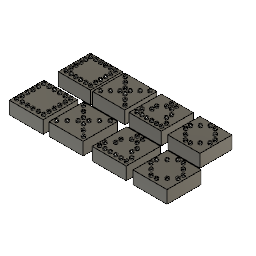
BrailleResearchShapes (Autodesk Fusion 360 design; units mm, degrees)
Autodesk Fusion 360 part; units mm, degrees
(part 1 of 2)
sketch "Sketch1" plane through (0, 0, 0) normal (0, 0, 1) x (1, 0, 0)
  circle A0 centre (3.4, 9.3) radius 0.75
  circle A1 centre (5.7, 9.2955) radius 0.75
  circle A2 centre (3.4, 7) radius 0.75
  circle A3 centre (5.7, 7) radius 0.75
  circle A4 centre (3.4, 4.7) radius 0.75
  circle A5 centre (5.7, 4.7) radius 0.75
  circle A6 centre (8, 9.3) radius 0.75
  circle A7 centre (10.3, 9.2955) radius 0.75
  circle A8 centre (10.3, 7) radius 0.75
  circle A9 centre (8, 7) radius 0.75
  circle A10 centre (10.3, 4.7) radius 0.75
  circle A11 centre (8, 4.7) radius 0.75
  circle A12 centre (12.6, 9.3) radius 0.75
  circle A13 centre (14.9, 7) radius 0.75
  circle A14 centre (14.9, 9.2955) radius 0.75
  circle A15 centre (12.6, 7) radius 0.75
  circle A16 centre (12.6, 4.7) radius 0.75
  circle A17 centre (14.9, 4.7) radius 0.75
  circle A18 centre (3.4, 2.4) radius 0.75
  circle A19 centre (5.7, 2.3955) radius 0.75
  circle A20 centre (5.7, 0.1) radius 0.75
  circle A21 centre (8, 0) radius 0.75
  circle A22 centre (8, 2.3) radius 0.75
  circle A23 centre (3.4, 0.1) radius 0.75
  circle A24 centre (10.3, 2.2955) radius 0.75
  circle A25 centre (5.7, -2.2) radius 0.75
  circle A26 centre (12.6, 2.3) radius 0.75
  circle A27 centre (12.6, 0) radius 0.75
  circle A28 centre (10.3, -2.3) radius 0.75
  circle A29 centre (10.3, 0) radius 0.75
  circle A30 centre (3.4, -2.2) radius 0.75
  circle A31 centre (8, -2.3) radius 0.75
  circle A32 centre (14.9, 0) radius 0.75
  circle A33 centre (12.6, -2.3) radius 0.75
  circle A34 centre (14.9, -2.3) radius 0.75
  circle A35 centre (14.9, 2.2955) radius 0.75
  line L0 (1.5, 11) -> (16.5, 11)
  line L1 (16.5, 11) -> (16.5, -4)
  line L2 (16.5, -4) -> (1.5, -4)
  line L3 (1.5, -4) -> (1.5, 11)
  line L4 (17.5, 11) -> (32.5, 11)
  circle A36 centre (28.6, 9.3) radius 0.75
  circle A37 centre (26.3, 9.2955) radius 0.75
  circle A38 centre (24, 7) radius 0.75
  circle A39 centre (21.7, 9.2955) radius 0.75
  circle A40 centre (19.4, 9.3) radius 0.75
  circle A41 centre (19.4, 7) radius 0.75
  circle A42 centre (21.7, 7) radius 0.75
  circle A43 centre (28.6, 7) radius 0.75
  circle A44 centre (30.9, 7) radius 0.75
  line L5 (32.5, 11) -> (32.5, -4)
  circle A45 centre (30.9, 2.2955) radius 0.75
  circle A46 centre (30.9, 0) radius 0.75
  circle A47 centre (30.9, -2.3) radius 0.75
  line L6 (32.5, -4) -> (17.5, -4)
  line L7 (17.5, -4) -> (17.5, 11)
  circle A48 centre (19.4, 2.4) radius 0.75
  circle A49 centre (21.7, 2.3955) radius 0.75
  circle A50 centre (19.4, 4.7) radius 0.75
  circle A51 centre (24, 9.3) radius 0.75
  circle A52 centre (21.7, 4.7) radius 0.75
  circle A53 centre (24, 4.7) radius 0.75
  circle A54 centre (24, 2.3) radius 0.75
  circle A55 centre (26.3, 7) radius 0.75
  circle A56 centre (30.9, 9.2955) radius 0.75
  circle A57 centre (28.6, 4.7) radius 0.75
  circle A58 centre (26.3, 4.7) radius 0.75
  circle A59 centre (26.3, 2.2955) radius 0.75
  circle A60 centre (30.9, 4.7) radius 0.75
  circle A61 centre (28.6, 2.3) radius 0.75
  circle A62 centre (28.6, 0) radius 0.75
  circle A63 centre (26.3, 0) radius 0.75
  circle A64 centre (26.3, -2.3) radius 0.75
  circle A65 centre (28.6, -2.3) radius 0.75
  circle A66 centre (21.7, 0.1) radius 0.75
  circle A67 centre (24, 0) radius 0.75
  circle A68 centre (24, -2.3) radius 0.75
  circle A69 centre (21.7, -2.2) radius 0.75
  circle A70 centre (19.4, 0.1) radius 0.75
  circle A71 centre (19.4, -2.2) radius 0.75
  line L8 (34.5, 11) -> (49.5, 11)
  line L9 (49.5, 11) -> (49.5, -4)
  circle A72 centre (47.9, 9.2955) radius 0.75
  circle A73 centre (45.6, 9.3) radius 0.75
  circle A74 centre (45.6, 7) radius 0.75
  circle A75 centre (45.6, 4.7) radius 0.75
  circle A76 centre (45.6, 2.3) radius 0.75
  circle A77 centre (45.6, 0) radius 0.75
  circle A78 centre (45.6, -2.3) radius 0.75
  line L10 (49.5, -4) -> (34.5, -4)
  circle A79 centre (41, -2.3) radius 0.75
  circle A80 centre (38.7, -2.2) radius 0.75
  circle A81 centre (36.4, -2.2) radius 0.75
  line L11 (34.5, -4) -> (34.5, 11)
  circle A82 centre (36.4, 0.1) radius 0.75
  circle A83 centre (38.7, 2.3955) radius 0.75
  circle A84 centre (36.4, 2.4) radius 0.75
  circle A85 centre (36.4, 4.7) radius 0.75
  circle A86 centre (36.4, 7) radius 0.75
  circle A87 centre (36.4, 9.3) radius 0.75
  circle A88 centre (38.7, 9.2955) radius 0.75
  circle A89 centre (41, 9.3) radius 0.75
  circle A90 centre (43.3, 9.2955) radius 0.75
  circle A91 centre (43.3, 7) radius 0.75
  circle A92 centre (41, 7) radius 0.75
  circle A93 centre (41, 4.7) radius 0.75
  circle A94 centre (38.7, 7) radius 0.75
  circle A95 centre (38.7, 4.7) radius 0.75
  circle A96 centre (43.3, 4.7) radius 0.75
  circle A97 centre (47.9, 7) radius 0.75
  circle A98 centre (47.9, 4.7) radius 0.75
  circle A99 centre (47.9, 2.2955) radius 0.75
  circle A100 centre (47.9, 0) radius 0.75
  circle A101 centre (47.9, -2.3) radius 0.75
  circle A102 centre (43.3, -2.3) radius 0.75
  circle A103 centre (43.3, 0) radius 0.75
  circle A104 centre (43.3, 2.2955) radius 0.75
  circle A105 centre (41, 0) radius 0.75
  circle A106 centre (41, 2.3) radius 0.75
  circle A107 centre (38.7, 0.1) radius 0.75
  circle A108 centre (3.2346, -12.4941) radius 0.75
  circle A109 centre (5.7346, -12.4941) radius 0.75
  circle A110 centre (5.7346, -14.9941) radius 0.75
  circle A111 centre (3.2346, -14.9941) radius 0.75
  circle A112 centre (3.2346, -17.4941) radius 0.75
  circle A113 centre (5.7346, -17.4941) radius 0.75
  circle A114 centre (8.2346, -12.4941) radius 0.75
  circle A115 centre (10.7346, -14.9941) radius 0.75
  circle A116 centre (10.7346, -17.4941) radius 0.75
  circle A117 centre (8.2346, -17.4941) radius 0.75
  circle A118 centre (8.2346, -14.9941) radius 0.75
  circle A119 centre (10.7346, -12.4941) radius 0.75
  circle A120 centre (13.2346, -12.4941) radius 0.75
  circle A121 centre (13.2346, -14.9941) radius 0.75
  circle A122 centre (13.2346, -17.4941) radius 0.75
  circle A123 centre (15.7346, -17.4941) radius 0.75
  circle A124 centre (15.7346, -14.9941) radius 0.75
  circle A125 centre (15.7346, -12.4941) radius 0.75
  circle A126 centre (3.2346, -19.9941) radius 0.75
  circle A127 centre (5.7346, -19.9941) radius 0.75
  circle A128 centre (8.2346, -22.4941) radius 0.75
  circle A129 centre (5.7346, -24.9941) radius 0.75
  circle A130 centre (5.7346, -22.4941) radius 0.75
  circle A131 centre (8.2346, -19.9941) radius 0.75
  circle A132 centre (3.2346, -22.4941) radius 0.75
  circle A133 centre (3.2346, -24.9941) radius 0.75
  circle A134 centre (10.7346, -19.9941) radius 0.75
  circle A135 centre (10.7346, -22.4941) radius 0.75
  circle A136 centre (8.2346, -24.9941) radius 0.75
  circle A137 centre (10.7346, -24.9941) radius 0.75
  circle A138 centre (13.2346, -19.9941) radius 0.75
  circle A139 centre (15.7346, -19.9941) radius 0.75
  circle A140 centre (13.2346, -22.4941) radius 0.75
  circle A141 centre (13.2346, -24.9941) radius 0.75
  circle A142 centre (15.7346, -22.4941) radius 0.75
  circle A143 centre (15.7346, -24.9941) radius 0.75
  line L12 (17.4146, -10.7288) -> (17.4146, -26.9182)
  line L13 (1.5963, -10.7288) -> (17.4146, -10.7288)
  line L14 (17.4146, -26.9182) -> (1.5963, -26.9182)
  line L15 (1.5963, -26.9182) -> (1.5963, -10.7288)
  line L16 (19.5963, -10.2888) -> (35.4146, -10.2888)
  line L17 (19.5963, -26.3316) -> (19.5963, -10.2888)
  circle A144 centre (21.2346, -11.9941) radius 0.75
  circle A145 centre (23.7346, -11.9941) radius 0.75
  circle A146 centre (21.2346, -16.9941) radius 0.75
  circle A147 centre (23.7346, -14.4941) radius 0.75
  circle A148 centre (26.2346, -11.9941) radius 0.75
  circle A149 centre (26.2346, -14.4941) radius 0.75
  circle A150 centre (23.7346, -16.9941) radius 0.75
  circle A151 centre (21.2346, -21.9941) radius 0.75
  circle A152 centre (23.7346, -19.4941) radius 0.75
  circle A153 centre (28.7346, -14.4941) radius 0.75
  circle A154 centre (26.2346, -16.9941) radius 0.75
  circle A155 centre (23.7346, -21.9941) radius 0.75
  circle A156 centre (28.7346, -16.9941) radius 0.75
  circle A157 centre (33.7346, -11.9941) radius 0.75
  circle A158 centre (31.2346, -14.4941) radius 0.75
  circle A159 centre (26.2346, -19.4941) radius 0.75
  line L18 (35.4146, -26.3316) -> (19.5963, -26.3316)
  circle A160 centre (23.7346, -24.4941) radius 0.75
  line L19 (35.4146, -10.2888) -> (35.4146, -26.3316)
  circle A161 centre (33.7346, -19.4941) radius 0.75
  circle A162 centre (31.2346, -24.4941) radius 0.75
  circle A163 centre (28.7346, -19.4941) radius 0.75
  circle A164 centre (33.7346, -14.4941) radius 0.75
  circle A165 centre (31.2346, -16.9941) radius 0.75
  circle A166 centre (31.2346, -19.4941) radius 0.75
  circle A167 centre (28.7346, -24.4941) radius 0.75
  circle A168 centre (31.2346, -21.9941) radius 0.75
  circle A169 centre (33.7346, -16.9941) radius 0.75
  circle A170 centre (33.7346, -21.9941) radius 0.75
  circle A171 centre (33.7346, -24.4941) radius 0.75
  circle A172 centre (26.2346, -24.4941) radius 0.75
  circle A173 centre (26.2346, -21.9941) radius 0.75
  circle A174 centre (28.7346, -21.9941) radius 0.75
  circle A175 centre (21.2346, -24.4941) radius 0.75
  circle A176 centre (21.2346, -19.4941) radius 0.75
  circle A177 centre (21.2346, -14.4941) radius 0.75
  circle A178 centre (31.2346, -11.9941) radius 0.75
  circle A179 centre (28.7346, -11.9941) radius 0.75
  line L20 (19.5963, -10.2888) -> (35.4146, -10.2888)
  line L21 (19.5963, -25.8184) -> (19.5963, -10.2888)
  circle A180 centre (21.2346, -19.4941) radius 0.75
  circle A181 centre (23.7346, -19.4941) radius 0.75
  circle A182 centre (21.2346, -24.4941) radius 0.75
  circle A183 centre (23.7346, -24.4941) radius 0.75
  circle A184 centre (23.7346, -21.9941) radius 0.75
  circle A185 centre (26.2346, -21.9941) radius 0.75
  circle A186 centre (26.2346, -24.4941) radius 0.75
  circle A187 centre (28.7346, -24.4941) radius 0.75
  circle A188 centre (33.7346, -19.4941) radius 0.75
  circle A189 centre (31.2346, -21.9941) radius 0.75
  circle A190 centre (28.7346, -21.9941) radius 0.75
  circle A191 centre (31.2346, -24.4941) radius 0.75
  circle A192 centre (33.7346, -24.4941) radius 0.75
  circle A193 centre (33.7346, -21.9941) radius 0.75
  line L22 (35.4146, -10.2888) -> (35.4146, -25.8184)
  circle A194 centre (31.2346, -19.4941) radius 0.75
  circle A195 centre (28.7346, -19.4941) radius 0.75
  circle A196 centre (26.2346, -19.4941) radius 0.75
  circle A197 centre (21.2346, -21.9941) radius 0.75
  line L23 (39.5963, -10.2888) -> (55.4146, -10.2888)
  line L24 (39.5963, -10.2888) -> (55.4146, -10.2888)
  circle A198 centre (41.2346, -11.9941) radius 0.75
  circle A199 centre (41.2346, -14.4941) radius 0.75
  line L25 (39.5963, -25.8184) -> (39.5963, -10.2888)
  line L26 (39.5963, -26.2583) -> (39.5963, -10.2888)
  circle A200 centre (43.7346, -14.4941) radius 0.75
  circle A201 centre (43.7346, -19.4941) radius 0.75
  circle A202 centre (43.7346, -19.4941) radius 0.75
  circle A203 centre (41.2346, -24.4941) radius 0.75
  circle A204 centre (41.2346, -24.4941) radius 0.75
  line L27 (55.4146, -26.2583) -> (39.5963, -26.2583)
  circle A205 centre (43.7346, -24.4941) radius 0.75
  circle A206 centre (43.7346, -24.4941) radius 0.75
  circle A207 centre (48.7346, -16.9941) radius 0.75
  circle A208 centre (46.2346, -19.4941) radius 0.75
  circle A209 centre (46.2346, -19.4941) radius 0.75
  circle A210 centre (46.2346, -16.9941) radius 0.75
  circle A211 centre (43.7346, -16.9941) radius 0.75
  circle A212 centre (41.2346, -21.9941) radius 0.75
  circle A213 centre (41.2346, -21.9941) radius 0.75
  circle A214 centre (41.2346, -19.4941) radius 0.75
  circle A215 centre (41.2346, -19.4941) radius 0.75
  circle A216 centre (43.7346, -11.9941) radius 0.75
  circle A217 centre (41.2346, -16.9941) radius 0.75
  circle A218 centre (46.2346, -11.9941) radius 0.75
  circle A219 centre (43.7346, -21.9941) radius 0.75
  circle A220 centre (43.7346, -21.9941) radius 0.75
  circle A221 centre (51.2346, -16.9941) radius 0.75
  line L28 (55.4146, -10.2888) -> (55.4146, -26.2583)
  line L29 (55.4146, -10.2888) -> (55.4146, -25.8184)
  circle A222 centre (53.7346, -24.4941) radius 0.75
  circle A223 centre (53.7346, -24.4941) radius 0.75
  circle A224 centre (53.7346, -21.9941) radius 0.75
  circle A225 centre (53.7346, -21.9941) radius 0.75
  circle A226 centre (53.7346, -11.9941) radius 0.75
  circle A227 centre (53.7346, -16.9941) radius 0.75
  circle A228 centre (53.7346, -19.4941) radius 0.75
  circle A229 centre (53.7346, -19.4941) radius 0.75
  circle A230 centre (53.7346, -14.4941) radius 0.75
  circle A231 centre (51.2346, -19.4941) radius 0.75
  circle A232 centre (51.2346, -19.4941) radius 0.75
  circle A233 centre (51.2346, -21.9941) radius 0.75
  circle A234 centre (51.2346, -21.9941) radius 0.75
  circle A235 centre (51.2346, -14.4941) radius 0.75
  circle A236 centre (51.2346, -11.9941) radius 0.75
  circle A237 centre (48.7346, -14.4941) radius 0.75
  circle A238 centre (48.7346, -11.9941) radius 0.75
  circle A239 centre (46.2346, -14.4941) radius 0.75
  circle A240 centre (48.7346, -19.4941) radius 0.75
  circle A241 centre (48.7346, -19.4941) radius 0.75
  circle A242 centre (48.7346, -21.9941) radius 0.75
  circle A243 centre (48.7346, -21.9941) radius 0.75
  circle A244 centre (48.7346, -24.4941) radius 0.75
  circle A245 centre (48.7346, -24.4941) radius 0.75
  circle A246 centre (46.2346, -24.4941) radius 0.75
  circle A247 centre (46.2346, -24.4941) radius 0.75
  circle A248 centre (46.2346, -21.9941) radius 0.75
  circle A249 centre (46.2346, -21.9941) radius 0.75
  circle A250 centre (51.2346, -24.4941) radius 0.75
  circle A251 centre (51.2346, -24.4941) radius 0.75
  circle A252 centre (72.7346, -19.4941) radius 0.75
  circle A253 centre (70.2346, -19.4941) radius 0.75
  circle A254 centre (70.2346, -21.9941) radius 0.75
  circle A255 centre (67.7346, -19.4941) radius 0.75
  circle A256 centre (67.7346, -21.9941) radius 0.75
  circle A257 centre (70.2346, -24.4941) radius 0.75
  circle A258 centre (62.7346, -19.4941) radius 0.75
  circle A259 centre (65.2346, -19.4941) radius 0.75
  circle A260 centre (65.2346, -24.4941) radius 0.75
  circle A261 centre (72.7346, -21.9941) radius 0.75
  circle A262 centre (72.7346, -21.9941) radius 0.75
  circle A263 centre (62.7346, -21.9941) radius 0.75
  circle A264 centre (70.2346, -19.4941) radius 0.75
  circle A265 centre (65.2346, -24.4941) radius 0.75
  circle A266 centre (65.2346, -21.9941) radius 0.75
  circle A267 centre (70.2346, -24.4941) radius 0.75
  circle A268 centre (62.7346, -24.4941) radius 0.75
  circle A269 centre (72.7346, -19.4941) radius 0.75
  circle A270 centre (72.7346, -24.4941) radius 0.75
  circle A271 centre (72.7346, -11.9941) radius 0.75
  circle A272 centre (70.2346, -11.9941) radius 0.75
  circle A273 centre (65.2346, -14.4941) radius 0.75
  circle A274 centre (65.2346, -16.9941) radius 0.75
  circle A275 centre (62.7346, -16.9941) radius 0.75
  circle A276 centre (70.2346, -16.9941) radius 0.75
  circle A277 centre (65.2346, -11.9941) radius 0.75
  circle A278 centre (72.7346, -16.9941) radius 0.75
  circle A279 centre (67.7346, -14.4941) radius 0.75
  circle A280 centre (62.7346, -11.9941) radius 0.75
  circle A281 centre (62.7346, -14.4941) radius 0.75
  circle A282 centre (67.7346, -16.9941) radius 0.75
  circle A283 centre (67.7346, -11.9941) radius 0.75
  circle A284 centre (72.7346, -14.4941) radius 0.75
  circle A285 centre (70.2346, -14.4941) radius 0.75
  circle A286 centre (65.2346, -19.4941) radius 0.75
  circle A287 centre (62.7346, -19.4941) radius 0.75
  circle A288 centre (62.7346, -24.4941) radius 0.75
  circle A289 centre (72.7346, -24.4941) radius 0.75
  line L30 (58.5963, -10.2888) -> (74.4146, -10.2888)
  circle A290 centre (70.2346, -21.9941) radius 0.75
  line L31 (74.4146, -26.2583) -> (58.5963, -26.2583)
  circle A291 centre (67.7346, -24.4941) radius 0.75
  circle A292 centre (67.7346, -24.4941) radius 0.75
  circle A293 centre (62.7346, -21.9941) radius 0.75
  circle A294 centre (67.7346, -19.4941) radius 0.75
  circle A295 centre (67.7346, -21.9941) radius 0.75
  circle A296 centre (65.2346, -21.9941) radius 0.75
  line L32 (58.5963, -10.2888) -> (74.4146, -10.2888)
  line L33 (74.4146, -10.2888) -> (74.4146, -25.8184)
  line L34 (74.4146, -10.2888) -> (74.4146, -26.2583)
  circle A297 centre (60.2346, -11.9941) radius 0.75
  line L35 (58.5963, -25.8184) -> (58.5963, -10.2888)
  circle A298 centre (60.2346, -14.4941) radius 0.75
  line L36 (58.5963, -26.2583) -> (58.5963, -10.2888)
  circle A299 centre (60.2346, -16.9941) radius 0.75
  circle A300 centre (60.2346, -24.4941) radius 0.75
  circle A301 centre (60.2346, -21.9941) radius 0.75
  circle A302 centre (60.2346, -24.4941) radius 0.75
  circle A303 centre (60.2346, -21.9941) radius 0.75
  circle A304 centre (60.2346, -19.4941) radius 0.75
  circle A305 centre (60.2346, -19.4941) radius 0.75
  circle A306 centre (56.7, 7) radius 0.75
  circle A307 centre (65.9, 9.2955) radius 0.75
  circle A308 centre (56.7, 4.7) radius 0.75
  line L37 (67.5, -4) -> (52.5, -4)
  circle A309 centre (63.6, 7) radius 0.75
  circle A310 centre (65.9, 2.2955) radius 0.75
  line L38 (52.5, 11) -> (67.5, 11)
  circle A311 centre (65.9, -2.3) radius 0.75
  circle A312 centre (63.6, 9.3) radius 0.75
  circle A313 centre (54.4, -2.2) radius 0.75
  circle A314 centre (56.7, 2.3955) radius 0.75
  circle A315 centre (59, 9.3) radius 0.75
  circle A316 centre (63.6, -2.3) radius 0.75
  circle A317 centre (59, -2.3) radius 0.75
  circle A318 centre (65.9, 7) radius 0.75
  circle A319 centre (61.3, 7) radius 0.75
  circle A320 centre (59, 2.3) radius 0.75
  circle A321 centre (61.3, -2.3) radius 0.75
  circle A322 centre (56.7, -2.2) radius 0.75
  circle A323 centre (59, 4.7) radius 0.75
  circle A324 centre (59, 0) radius 0.75
  line L39 (67.5, 11) -> (67.5, -4)
  circle A325 centre (63.6, 4.7) radius 0.75
  circle A326 centre (65.9, 0) radius 0.75
  circle A327 centre (63.6, 0) radius 0.75
  line L40 (52.5, -4) -> (52.5, 11)
  circle A328 centre (54.4, 9.3) radius 0.75
  circle A329 centre (54.4, 4.7) radius 0.75
  circle A330 centre (65.9, 4.7) radius 0.75
  circle A331 centre (54.4, 2.4) radius 0.75
  circle A332 centre (54.4, 7) radius 0.75
  circle A333 centre (63.6, 2.3) radius 0.75
  circle A334 centre (54.4, 0.1) radius 0.75
  circle A335 centre (61.3, 4.7) radius 0.75
  circle A336 centre (61.3, 2.2955) radius 0.75
  circle A337 centre (56.7, 0.1) radius 0.75
  circle A338 centre (59, 7) radius 0.75
  circle A339 centre (61.3, 0) radius 0.75
  circle A340 centre (56.7, 9.2955) radius 0.75
  circle A341 centre (61.3, 9.2955) radius 0.75
  dimension "d1" = 1.5
  dimension "d2" = 1.5
  dimension "d4" = 1.5
  dimension "d5" = 1.5
  dimension "d6" = 1.5
  dimension "d7" = 1.5
  dimension "d8" = 2.3
  dimension "d9" = 2.3
  dimension "d10" = 2.3
  dimension "d11" = 1.5
  dimension "d12" = 1.5
  dimension "d13" = 1.5
  dimension "d14" = 1.5
  dimension "d15" = 1.5
  dimension "d16" = 1.5
  dimension "d17" = 2.3
  dimension "d18" = 2.3
  dimension "d19" = 2.3
  dimension "d20" = 1.5
  dimension "d21" = 1.5
  dimension "d22" = 1.5
  dimension "d23" = 1.5
  dimension "d24" = 1.5
  dimension "d25" = 1.5
  dimension "d26" = 2.3
  dimension "d27" = 2.3
  dimension "d28" = 2.3
  dimension "d29" = 2.3
  dimension "d30" = 2.3
  dimension "d31" = 1.5
  dimension "d32" = 1.5
  dimension "d33" = 1.5
  dimension "d34" = 1.5
  dimension "d35" = 1.5
  dimension "d36" = 1.5
  dimension "d37" = 2.3
  dimension "d38" = 2.3
  dimension "d39" = 2.3
  dimension "d40" = 1.5
  dimension "d41" = 1.5
  dimension "d42" = 1.5
  dimension "d43" = 1.5
  dimension "d44" = 1.5
  dimension "d45" = 1.5
  dimension "d46" = 2.3
  dimension "d47" = 2.3
  dimension "d48" = 2.3
  dimension "d49" = 1.5
  dimension "d50" = 1.5
  dimension "d51" = 1.5
  dimension "d52" = 1.5
  dimension "d53" = 1.5
  dimension "d54" = 1.5
  dimension "d55" = 2.3
  dimension "d56" = 2.3
  dimension "d57" = 2.3
  dimension "d58" = 2.3
  dimension "d59" = 2.3
  dimension "d60" = 2.3
  dimension "d61" = 1.5
  dimension "d62" = 1.5
  dimension "d63" = 1.5
  dimension "d64" = 1.5
  dimension "d65" = 1.5
  dimension "d66" = 1.5
  dimension "d67" = 2.3
  dimension "d68" = 2.3
  dimension "d69" = 2.3
  dimension "d70" = 1.5
  dimension "d71" = 1.5
  dimension "d72" = 1.5
  dimension "d73" = 1.5
  dimension "d74" = 1.5
  dimension "d75" = 1.5
  dimension "d76" = 2.3
  dimension "d77" = 2.3
  dimension "d78" = 2.3
  dimension "d79" = 1.5
  dimension "d80" = 1.5
  dimension "d81" = 1.5
  dimension "d82" = 1.5
  dimension "d83" = 1.5
  dimension "d84" = 1.5
  dimension "d85" = 2.3
  dimension "d86" = 2.3
  dimension "d87" = 2.3
  dimension "d88" = 2.3
  dimension "d89" = 2.3
  dimension "d90" = 1.5
  dimension "d91" = 1.5
  dimension "d92" = 1.5
  dimension "d93" = 1.5
  dimension "d94" = 1.5
  dimension "d95" = 1.5
  dimension "d96" = 2.3
  dimension "d97" = 2.3
  dimension "d98" = 2.3
  dimension "d99" = 1.5
  dimension "d100" = 1.5
  dimension "d101" = 1.5
  dimension "d102" = 1.5
  dimension "d103" = 1.5
  dimension "d104" = 1.5
  dimension "d105" = 2.3
  dimension "d106" = 2.3
  dimension "d107" = 2.3
  dimension "d108" = 1.5
  dimension "d109" = 1.5
  dimension "d110" = 1.5
  dimension "d111" = 1.5
  dimension "d112" = 1.5
  dimension "d113" = 1.5
  dimension "d114" = 2.3
  dimension "d115" = 2.3
  dimension "d116" = 2.3
  dimension "d117" = 2.3
  dimension "d118" = 2.3
  dimension "d119" = 2.3
  dimension "d120" = 1.5
  dimension "d121" = 1.5
  dimension "d122" = 1.5
  dimension "d123" = 1.5
  dimension "d124" = 1.5
  dimension "d125" = 1.5
  dimension "d126" = 2.3
  dimension "d127" = 2.3
  dimension "d128" = 2.3
  dimension "d129" = 1.5
  dimension "d130" = 1.5
  dimension "d131" = 1.5
  dimension "d132" = 1.5
  dimension "d133" = 1.5
  dimension "d134" = 1.5
  dimension "d135" = 2.3
  dimension "d136" = 2.3
  dimension "d137" = 2.3
  dimension "d138" = 1.5
  dimension "d139" = 1.5
  dimension "d140" = 1.5
  dimension "d141" = 1.5
  dimension "d142" = 1.5
  dimension "d143" = 1.5
  dimension "d144" = 2.3
  dimension "d145" = 2.3
  dimension "d146" = 2.3
  dimension "d147" = 2.3
  dimension "d148" = 2.3
  dimension "d149" = 1.5
  dimension "d150" = 1.5
  dimension "d151" = 1.5
  dimension "d152" = 1.5
  dimension "d153" = 1.5
  dimension "d154" = 1.5
  dimension "d155" = 2.3
  dimension "d156" = 2.3
  dimension "d157" = 2.3
  dimension "d158" = 1.5
  dimension "d159" = 1.5
  dimension "d160" = 1.5
  dimension "d161" = 1.5
  dimension "d162" = 1.5
  dimension "d163" = 1.5
  dimension "d164" = 2.3
  dimension "d165" = 2.3
  dimension "d166" = 2.3
  dimension "d167" = 1.5
  dimension "d168" = 1.5
  dimension "d169" = 1.5
  dimension "d170" = 1.5
  dimension "d171" = 1.5
  dimension "d172" = 1.5
  dimension "d173" = 2.3
  dimension "d174" = 2.3
  dimension "d175" = 2.3
  dimension "d176" = 2.3
  dimension "d177" = 2.3
  dimension "d178" = 2.3
  dimension "d199" = 1.5
  dimension "d200" = 1.5
  dimension "d201" = 1.5
  dimension "d202" = 1.5
  dimension "d203" = 1.5
  dimension "d204" = 1.5
  dimension "d208" = 2.5
  dimension "d209" = 2.5
  dimension "d210" = 2.5
  dimension "d211" = 1.5
  dimension "d212" = 1.5
  dimension "d213" = 1.5
  dimension "d214" = 1.5
  dimension "d215" = 1.5
  dimension "d216" = 1.5
  dimension "d217" = 2.5
  dimension "d218" = 2.5
  dimension "d219" = 2.5
  dimension "d220" = 1.5
  dimension "d221" = 1.5
  dimension "d222" = 1.5
  dimension "d223" = 1.5
  dimension "d224" = 1.5
  dimension "d225" = 1.5
  dimension "d226" = 2.5
  dimension "d227" = 2.5
  dimension "d228" = 2.5
  dimension "d229" = 2.5
  dimension "d230" = 2.5
  dimension "d231" = 1.5
  dimension "d232" = 1.5
  dimension "d233" = 1.5
  dimension "d234" = 1.5
  dimension "d235" = 1.5
  dimension "d236" = 1.5
  dimension "d237" = 2.5
  dimension "d238" = 2.5
  dimension "d239" = 2.5
  dimension "d240" = 1.5
  dimension "d241" = 1.5
  dimension "d242" = 1.5
  dimension "d243" = 1.5
  dimension "d244" = 1.5
  dimension "d245" = 1.5
  dimension "d246" = 2.5
  dimension "d247" = 2.5
  dimension "d248" = 2.5
  dimension "d249" = 1.5
  dimension "d250" = 1.5
  dimension "d251" = 1.5
  dimension "d252" = 1.5
  dimension "d253" = 1.5
  dimension "d254" = 1.5
  dimension "d255" = 2.5
  dimension "d256" = 2.5
  dimension "d257" = 2.5
  dimension "d258" = 2.5
  dimension "d259" = 2.5
  dimension "d260" = 2.5
  dimension "d261" = 1.5
  dimension "d262" = 1.5
  dimension "d263" = 1.5
  dimension "d264" = 1.5
  dimension "d265" = 1.5
  dimension "d266" = 1.5
  dimension "d267" = 2.5
  dimension "d268" = 2.5
  dimension "d269" = 2.5
  dimension "d270" = 1.5
  dimension "d271" = 1.5
  dimension "d272" = 1.5
  dimension "d273" = 1.5
  dimension "d274" = 1.5
  dimension "d275" = 1.5
  dimension "d276" = 2.5
  dimension "d277" = 2.5
  dimension "d278" = 2.5
  dimension "d279" = 1.5
  dimension "d280" = 1.5
  dimension "d281" = 1.5
  dimension "d282" = 1.5
  dimension "d283" = 1.5
  dimension "d284" = 1.5
  dimension "d285" = 2.5
  dimension "d286" = 2.5
  dimension "d287" = 2.5
  dimension "d288" = 2.5
  dimension "d289" = 2.5
  dimension "d290" = 1.5
  dimension "d291" = 1.5
  dimension "d292" = 1.5
  dimension "d293" = 1.5
  dimension "d294" = 1.5
  dimension "d295" = 1.5
  dimension "d296" = 2.5
  dimension "d297" = 2.5
  dimension "d298" = 2.5
  dimension "d299" = 1.5
  dimension "d300" = 1.5
  dimension "d301" = 1.5
  dimension "d302" = 1.5
  dimension "d303" = 1.5
  dimension "d304" = 1.5
  dimension "d305" = 2.5
  dimension "d306" = 2.5
  dimension "d307" = 2.5
  dimension "d308" = 1.5
  dimension "d309" = 1.5
  dimension "d310" = 1.5
  dimension "d311" = 1.5
  dimension "d312" = 1.5
  dimension "d313" = 1.5
  dimension "d314" = 2.5
  dimension "d315" = 2.5
  dimension "d316" = 2.5
  dimension "d317" = 2.5
  dimension "d318" = 2.5
  dimension "d319" = 2.5
  dimension "d349" = 1.5
  dimension "d350" = 1.5
  dimension "d351" = 1.5
  dimension "d352" = 1.5
  dimension "d353" = 1.5
  dimension "d354" = 1.5
  dimension "d355" = 2.5
  dimension "d356" = 2.5
  dimension "d357" = 2.5
  dimension "d358" = 1.5
  dimension "d359" = 1.5
  dimension "d360" = 1.5
  dimension "d361" = 1.5
  dimension "d362" = 1.5
  dimension "d363" = 1.5
  dimension "d364" = 2.5
  dimension "d365" = 2.5
  dimension "d366" = 2.5
  dimension "d367" = 1.5
  dimension "d368" = 1.5
  dimension "d369" = 1.5
  dimension "d370" = 1.5
  dimension "d371" = 1.5
  dimension "d372" = 1.5
  dimension "d373" = 2.5
  dimension "d374" = 2.5
  dimension "d375" = 2.5
  dimension "d376" = 2.5
  dimension "d377" = 2.5
  dimension "d408" = 1.5
  dimension "d409" = 1.5
  dimension "d410" = 1.5
  dimension "d411" = 1.5
  dimension "d412" = 1.5
  dimension "d413" = 1.5
  dimension "d414" = 2.5
  dimension "d415" = 2.5
  dimension "d416" = 2.5
  dimension "d417" = 1.5
  dimension "d418" = 1.5
  dimension "d419" = 1.5
  dimension "d420" = 1.5
  dimension "d421" = 1.5
  dimension "d422" = 1.5
  dimension "d423" = 2.5
  dimension "d424" = 2.5
  dimension "d425" = 2.5
  dimension "d426" = 1.5
  dimension "d427" = 1.5
  dimension "d428" = 1.5
  dimension "d429" = 1.5
  dimension "d430" = 1.5
  dimension "d431" = 1.5
  dimension "d432" = 2.5
  dimension "d433" = 2.5
  dimension "d434" = 2.5
  dimension "d435" = 2.5
  dimension "d436" = 2.5
  dimension "d438" = 1.5
  dimension "d439" = 1.5
  dimension "d440" = 1.5
  dimension "d441" = 1.5
  dimension "d442" = 1.5
  dimension "d443" = 1.5
  dimension "d444" = 2.5
  dimension "d445" = 2.5
  dimension "d446" = 2.5
  dimension "d447" = 1.5
  dimension "d448" = 1.5
  dimension "d449" = 1.5
  dimension "d450" = 1.5
  dimension "d451" = 1.5
  dimension "d452" = 1.5
  dimension "d453" = 2.5
  dimension "d454" = 2.5
  dimension "d455" = 2.5
  dimension "d456" = 1.5
  dimension "d457" = 1.5
  dimension "d458" = 1.5
  dimension "d459" = 1.5
  dimension "d460" = 1.5
  dimension "d461" = 1.5
  dimension "d462" = 2.5
  dimension "d463" = 2.5
  dimension "d464" = 2.5
  dimension "d465" = 2.5
  dimension "d466" = 2.5
  dimension "d467" = 1.5
  dimension "d468" = 1.5
  dimension "d469" = 1.5
  dimension "d470" = 1.5
  dimension "d471" = 1.5
  dimension "d472" = 1.5
  dimension "d473" = 2.5
  dimension "d474" = 2.5
  dimension "d475" = 2.5
  dimension "d476" = 1.5
  dimension "d477" = 1.5
  dimension "d478" = 1.5
  dimension "d479" = 1.5
  dimension "d480" = 1.5
  dimension "d481" = 1.5
  dimension "d482" = 2.5
  dimension "d483" = 2.5
  dimension "d484" = 2.5
  dimension "d485" = 1.5
  dimension "d486" = 1.5
  dimension "d487" = 1.5
  dimension "d488" = 1.5
  dimension "d489" = 1.5
  dimension "d490" = 1.5
  dimension "d491" = 2.5
  dimension "d492" = 2.5
  dimension "d493" = 2.5
  dimension "d494" = 2.5
  dimension "d495" = 2.5
  dimension "d496" = 2.5
  dimension "d503" = 1.5
  dimension "d504" = 1.5
  dimension "d505" = 1.5
  dimension "d506" = 1.5
  dimension "d507" = 1.5
  dimension "d508" = 1.5
  dimension "d509" = 2.5
  dimension "d510" = 2.5
  dimension "d511" = 2.5
  dimension "d512" = 1.5
  dimension "d513" = 1.5
  dimension "d514" = 1.5
  dimension "d515" = 1.5
  dimension "d516" = 1.5
  dimension "d517" = 1.5
  dimension "d518" = 2.5
  dimension "d519" = 2.5
  dimension "d520" = 2.5
  dimension "d521" = 1.5
  dimension "d522" = 1.5
  dimension "d523" = 1.5
  dimension "d524" = 1.5
  dimension "d525" = 1.5
  dimension "d526" = 1.5
  dimension "d527" = 2.5
  dimension "d528" = 2.5
  dimension "d529" = 2.5
  dimension "d530" = 2.5
  dimension "d531" = 2.5
  dimension "d532" = 1.5
  dimension "d533" = 1.5
  dimension "d534" = 1.5
  dimension "d535" = 1.5
  dimension "d536" = 1.5
  dimension "d537" = 1.5
  dimension "d538" = 2.5
  dimension "d539" = 2.5
  dimension "d540" = 2.5
  dimension "d541" = 1.5
  dimension "d542" = 1.5
  dimension "d543" = 1.5
  dimension "d544" = 1.5
  dimension "d545" = 1.5
  dimension "d546" = 1.5
  dimension "d547" = 2.5
  dimension "d548" = 2.5
  dimension "d549" = 2.5
  dimension "d550" = 1.5
  dimension "d551" = 1.5
  dimension "d552" = 1.5
  dimension "d553" = 1.5
  dimension "d554" = 1.5
  dimension "d555" = 1.5
  dimension "d556" = 2.5
  dimension "d557" = 2.5
  dimension "d558" = 2.5
  dimension "d559" = 2.5
  dimension "d560" = 2.5
  dimension "d561" = 1.5
  dimension "d562" = 1.5
  dimension "d563" = 1.5
  dimension "d564" = 1.5
  dimension "d565" = 1.5
  dimension "d566" = 1.5
  dimension "d567" = 2.5
  dimension "d568" = 2.5
  dimension "d569" = 2.5
  dimension "d570" = 1.5
  dimension "d571" = 1.5
  dimension "d572" = 1.5
  dimension "d573" = 1.5
  dimension "d574" = 1.5
  dimension "d575" = 1.5
  dimension "d576" = 2.5
  dimension "d577" = 2.5
  dimension "d578" = 2.5
  dimension "d579" = 1.5
  dimension "d580" = 1.5
  dimension "d581" = 1.5
  dimension "d582" = 1.5
  dimension "d583" = 1.5
  dimension "d584" = 1.5
  dimension "d585" = 2.5
  dimension "d586" = 2.5
  dimension "d587" = 2.5
  dimension "d588" = 2.5
  dimension "d589" = 2.5
  dimension "d590" = 2.5
  dimension "d591" = 1.5
  dimension "d592" = 1.5
  dimension "d593" = 1.5
  dimension "d594" = 1.5
  dimension "d595" = 1.5
  dimension "d596" = 1.5
  dimension "d597" = 2.3
  dimension "d598" = 2.3
  dimension "d599" = 2.3
  dimension "d600" = 1.5
  dimension "d601" = 1.5
  dimension "d602" = 1.5
  dimension "d603" = 1.5
  dimension "d604" = 1.5
  dimension "d605" = 1.5
  dimension "d606" = 2.3
  dimension "d607" = 2.3
  dimension "d608" = 2.3
  dimension "d609" = 1.5
  dimension "d610" = 1.5
  dimension "d611" = 1.5
  dimension "d612" = 1.5
  dimension "d613" = 1.5
  dimension "d614" = 1.5
  dimension "d615" = 2.3
  dimension "d616" = 2.3
  dimension "d617" = 2.3
  dimension "d618" = 2.3
  dimension "d619" = 2.3
  dimension "d620" = 1.5
  dimension "d621" = 1.5
  dimension "d622" = 1.5
  dimension "d623" = 1.5
  dimension "d624" = 1.5
  dimension "d625" = 1.5
  dimension "d626" = 2.3
  dimension "d627" = 2.3
  dimension "d628" = 2.3
  dimension "d629" = 1.5
  dimension "d630" = 1.5
  dimension "d631" = 1.5
  dimension "d632" = 1.5
  dimension "d633" = 1.5
  dimension "d634" = 1.5
  dimension "d635" = 2.3
  dimension "d636" = 2.3
  dimension "d637" = 2.3
  dimension "d638" = 1.5
  dimension "d639" = 1.5
  dimension "d640" = 1.5
  dimension "d641" = 1.5
  dimension "d642" = 1.5
  dimension "d643" = 1.5
  dimension "d644" = 2.3
  dimension "d645" = 2.3
  dimension "d646" = 2.3
  dimension "d647" = 2.3
  dimension "d648" = 2.3
  dimension "d649" = 2.3
  constraint vertical A1.centre A3.centre
  constraint vertical A3.centre A5.centre
  constraint horizontal A5.centre A4.centre
  constraint horizontal A3.centre A2.centre
  constraint vertical A7.centre A8.centre
  constraint vertical A10.centre A8.centre
  constraint horizontal A10.centre A11.centre
  constraint horizontal A8.centre A9.centre
  constraint vertical A13.centre A14.centre
  constraint vertical A13.centre A17.centre
  constraint horizontal A17.centre A16.centre
  constraint horizontal A13.centre A15.centre
  constraint vertical A19.centre A20.centre
  constraint vertical A25.centre A20.centre
  constraint horizontal A25.centre A30.centre
  constraint horizontal A20.centre A23.centre
  constraint vertical A29.centre A24.centre
  constraint vertical A29.centre A28.centre
  constraint horizontal A28.centre A31.centre
  constraint horizontal A29.centre A21.centre
  constraint vertical A35.centre A32.centre
  constraint vertical A32.centre A34.centre
  constraint horizontal A33.centre A34.centre
  constraint horizontal A27.centre A32.centre
  constraint horizontal L0
  constraint vertical L1
  constraint horizontal L2
  constraint vertical L3
  constraint vertical A39.centre A42.centre
  constraint vertical A52.centre A42.centre
  constraint horizontal A52.centre A50.centre
  constraint horizontal A42.centre A41.centre
  constraint vertical A55.centre A37.centre
  constraint vertical A55.centre A58.centre
  constraint horizontal A58.centre A53.centre
  constraint horizontal A55.centre A38.centre
  constraint vertical A56.centre A44.centre
  constraint vertical A44.centre A60.centre
  constraint horizontal A57.centre A60.centre
  constraint horizontal A43.centre A44.centre
  constraint vertical A49.centre A66.centre
  constraint vertical A69.centre A66.centre
  constraint horizontal A71.centre A69.centre
  constraint horizontal A66.centre A70.centre
  constraint vertical A63.centre A59.centre
  constraint vertical A63.centre A64.centre
  constraint horizontal A64.centre A68.centre
  constraint horizontal A63.centre A67.centre
  constraint vertical A45.centre A46.centre
  constraint vertical A47.centre A46.centre
  constraint horizontal A47.centre A65.centre
  constraint horizontal A62.centre A46.centre
  constraint horizontal L4
  constraint vertical L5
  constraint horizontal L6
  constraint vertical L7
  constraint vertical A94.centre A88.centre
  constraint vertical A94.centre A95.centre
  constraint horizontal A95.centre A85.centre
  constraint horizontal A94.centre A86.centre
  constraint vertical A91.centre A90.centre
  constraint vertical A91.centre A96.centre
  constraint horizontal A93.centre A96.centre
  constraint horizontal A92.centre A91.centre
  constraint vertical A72.centre A97.centre
  constraint vertical A97.centre A98.centre
  constraint horizontal A75.centre A98.centre
  constraint horizontal A74.centre A97.centre
  constraint vertical A83.centre A107.centre
  constraint vertical A80.centre A107.centre
  constraint horizontal A81.centre A80.centre
  constraint horizontal A107.centre A82.centre
  constraint vertical A104.centre A103.centre
  constraint vertical A102.centre A103.centre
  constraint horizontal A79.centre A102.centre
  constraint horizontal A105.centre A103.centre
  constraint vertical A99.centre A100.centre
  constraint vertical A101.centre A100.centre
  constraint horizontal A101.centre A78.centre
  constraint horizontal A77.centre A100.centre
  constraint horizontal L8
  constraint vertical L9
  constraint horizontal L10
  constraint vertical L11
  constraint vertical A109.centre A110.centre
  constraint vertical A113.centre A110.centre
  constraint horizontal A113.centre A112.centre
  constraint horizontal A110.centre A111.centre
  constraint vertical A111.centre A108.centre
  constraint horizontal A109.centre A108.centre
  constraint vertical A111.centre A112.centre
  constraint vertical A115.centre A119.centre
  constraint vertical A116.centre A115.centre
  constraint horizontal A116.centre A117.centre
  constraint horizontal A115.centre A118.centre
  constraint vertical A114.centre A118.centre
  constraint horizontal A114.centre A119.centre
  constraint vertical A118.centre A117.centre
  constraint vertical A125.centre A124.centre
  constraint vertical A123.centre A124.centre
  constraint horizontal A122.centre A123.centre
  constraint horizontal A124.centre A121.centre
  constraint vertical A120.centre A121.centre
  constraint horizontal A125.centre A120.centre
  constraint vertical A122.centre A121.centre
  constraint horizontal A119.centre A125.centre
  constraint horizontal A109.centre A114.centre
  constraint vertical A130.centre A127.centre
  constraint vertical A129.centre A130.centre
  constraint horizontal A129.centre A133.centre
  constraint horizontal A130.centre A132.centre
  constraint vertical A126.centre A132.centre
  constraint horizontal A126.centre A127.centre
  constraint vertical A132.centre A133.centre
  constraint vertical A134.centre A135.centre
  constraint vertical A137.centre A135.centre
  constraint horizontal A136.centre A137.centre
  constraint horizontal A135.centre A128.centre
  constraint vertical A131.centre A128.centre
  constraint horizontal A134.centre A131.centre
  constraint vertical A136.centre A128.centre
  constraint vertical A139.centre A142.centre
  constraint vertical A143.centre A142.centre
  constraint horizontal A143.centre A141.centre
  constraint horizontal A140.centre A142.centre
  constraint vertical A140.centre A138.centre
  constraint horizontal A138.centre A139.centre
  constraint vertical A140.centre A141.centre
  constraint horizontal A134.centre A139.centre
  constraint horizontal A131.centre A127.centre
  constraint horizontal L13
  constraint vertical L12
  constraint horizontal L14
  constraint vertical L15
  constraint vertical A147.centre A145.centre
  constraint vertical A150.centre A147.centre
  constraint horizontal A150.centre A146.centre
  constraint horizontal A147.centre A177.centre
  constraint vertical A144.centre A177.centre
  constraint horizontal A144.centre A145.centre
  constraint vertical A177.centre A146.centre
  constraint vertical A179.centre A153.centre
  constraint vertical A156.centre A153.centre
  constraint horizontal A154.centre A156.centre
  constraint horizontal A153.centre A149.centre
  constraint vertical A148.centre A149.centre
  constraint horizontal A179.centre A148.centre
  constraint vertical A154.centre A149.centre
  constraint vertical A157.centre A164.centre
  constraint vertical A169.centre A164.centre
  constraint horizontal A169.centre A165.centre
  constraint horizontal A158.centre A164.centre
  constraint vertical A158.centre A178.centre
  constraint horizontal A178.centre A157.centre
  constraint vertical A158.centre A165.centre
  constraint horizontal A179.centre A157.centre
  constraint horizontal A148.centre A145.centre
  constraint vertical A155.centre A152.centre
  constraint vertical A160.centre A155.centre
  constraint horizontal A160.centre A175.centre
  constraint horizontal A155.centre A151.centre
  constraint vertical A151.centre A176.centre
  constraint horizontal A152.centre A176.centre
  constraint vertical A151.centre A175.centre
  constraint vertical A174.centre A163.centre
  constraint vertical A174.centre A167.centre
  constraint horizontal A172.centre A167.centre
  constraint horizontal A174.centre A173.centre
  constraint vertical A159.centre A173.centre
  constraint horizontal A159.centre A163.centre
  constraint vertical A172.centre A173.centre
  constraint vertical A161.centre A170.centre
  constraint vertical A171.centre A170.centre
  constraint horizontal A171.centre A162.centre
  constraint horizontal A168.centre A170.centre
  constraint vertical A168.centre A166.centre
  constraint horizontal A166.centre A161.centre
  constraint vertical A168.centre A162.centre
  constraint horizontal A161.centre A163.centre
  constraint horizontal A152.centre A159.centre
  constraint horizontal L16
  constraint vertical L19
  constraint horizontal L18
  constraint vertical L17
  constraint vertical A152.centre A155.centre
  constraint horizontal A151.centre A155.centre
  constraint vertical A176.centre A151.centre
  constraint horizontal A176.centre A152.centre
  constraint vertical A167.centre A174.centre
  constraint horizontal A167.centre A172.centre
  constraint vertical A170.centre A171.centre
  constraint horizontal A162.centre A171.centre
  constraint horizontal A170.centre A168.centre
  constraint horizontal A161.centre A166.centre
  constraint horizontal A159.centre A152.centre
  constraint horizontal L20
  constraint vertical L22
  constraint vertical L21
  constraint vertical A201.centre A219.centre
  constraint vertical A205.centre A219.centre
  constraint horizontal A205.centre A203.centre
  constraint horizontal A212.centre A219.centre
  constraint vertical A214.centre A212.centre
  constraint horizontal A214.centre A201.centre
  constraint vertical A212.centre A203.centre
  constraint vertical A242.centre A240.centre
  constraint vertical A244.centre A242.centre
  constraint horizontal A244.centre A246.centre
  constraint horizontal A242.centre A248.centre
  constraint vertical A208.centre A248.centre
  constraint horizontal A208.centre A240.centre
  constraint vertical A246.centre A248.centre
  constraint vertical A228.centre A224.centre
  constraint vertical A224.centre A222.centre
  constraint horizontal A250.centre A222.centre
  constraint horizontal A224.centre A233.centre
  constraint vertical A233.centre A231.centre
  constraint horizontal A228.centre A231.centre
  constraint vertical A233.centre A250.centre
  constraint horizontal A228.centre A240.centre
  constraint horizontal A208.centre A201.centre
  constraint horizontal L24
  constraint vertical L29
  constraint vertical L25
  constraint vertical A200.centre A216.centre
  constraint vertical A200.centre A211.centre
  constraint horizontal A217.centre A211.centre
  constraint horizontal A199.centre A200.centre
  constraint vertical A199.centre A198.centre
  constraint horizontal A216.centre A198.centre
  constraint vertical A199.centre A217.centre
  constraint vertical A237.centre A238.centre
  constraint vertical A237.centre A207.centre
  constraint horizontal A207.centre A210.centre
  constraint horizontal A237.centre A239.centre
  constraint vertical A218.centre A239.centre
  constraint horizontal A238.centre A218.centre
  constraint vertical A239.centre A210.centre
  constraint vertical A226.centre A230.centre
  constraint vertical A227.centre A230.centre
  constraint horizontal A227.centre A221.centre
  constraint horizontal A235.centre A230.centre
  constraint vertical A235.centre A236.centre
  constraint horizontal A236.centre A226.centre
  constraint vertical A235.centre A221.centre
  constraint horizontal A226.centre A238.centre
  constraint horizontal A216.centre A218.centre
  constraint horizontal L23
  constraint vertical L28
  constraint horizontal L27
  constraint vertical L26
  constraint vertical A258.centre A263.centre
  constraint vertical A268.centre A263.centre
  constraint horizontal A268.centre A300.centre
  constraint horizontal A301.centre A263.centre
  constraint vertical A304.centre A301.centre
  constraint horizontal A304.centre A258.centre
  constraint vertical A301.centre A300.centre
  constraint vertical A256.centre A255.centre
  constraint vertical A256.centre A291.centre
  constraint horizontal A260.centre A291.centre
  constraint horizontal A256.centre A266.centre
  constraint vertical A266.centre A259.centre
  constraint horizontal A255.centre A259.centre
  constraint vertical A260.centre A266.centre
  constraint vertical A252.centre A261.centre
  constraint vertical A270.centre A261.centre
  constraint horizontal A257.centre A270.centre
  constraint horizontal A261.centre A254.centre
  constraint vertical A253.centre A254.centre
  constraint horizontal A253.centre A252.centre
  constraint vertical A257.centre A254.centre
  constraint horizontal A255.centre A252.centre
  constraint horizontal A258.centre A259.centre
  constraint horizontal L30
  constraint vertical L33
  constraint vertical L35
  constraint vertical A280.centre A281.centre
  constraint vertical A275.centre A281.centre
  constraint horizontal A275.centre A299.centre
  constraint horizontal A298.centre A281.centre
  constraint vertical A298.centre A297.centre
  constraint horizontal A297.centre A280.centre
  constraint vertical A298.centre A299.centre
  constraint vertical A279.centre A283.centre
  constraint vertical A282.centre A279.centre
  constraint horizontal A282.centre A274.centre
  constraint horizontal A273.centre A279.centre
  constraint vertical A273.centre A277.centre
  constraint horizontal A283.centre A277.centre
  constraint vertical A273.centre A274.centre
  constraint vertical A284.centre A271.centre
  constraint vertical A284.centre A278.centre
  constraint horizontal A278.centre A276.centre
  constraint horizontal A284.centre A285.centre
  constraint vertical A285.centre A272.centre
  constraint horizontal A272.centre A271.centre
  constraint vertical A285.centre A276.centre
  constraint horizontal A271.centre A283.centre
  constraint horizontal A280.centre A277.centre
  constraint vertical A301.centre A304.centre
  constraint horizontal A258.centre A304.centre
  constraint vertical A291.centre A256.centre
  constraint horizontal A291.centre A260.centre
  constraint vertical A259.centre A266.centre
  constraint horizontal A259.centre A255.centre
  constraint vertical A266.centre A260.centre
  constraint vertical A261.centre A270.centre
  constraint horizontal A270.centre A257.centre
  constraint vertical A254.centre A253.centre
  constraint horizontal A252.centre A253.centre
  constraint vertical A254.centre A257.centre
  constraint horizontal A252.centre A255.centre
  constraint horizontal A259.centre A258.centre
  constraint horizontal L32
  constraint vertical L34
  constraint horizontal L31
  constraint vertical L36
  constraint vertical A340.centre A306.centre
  constraint vertical A306.centre A308.centre
  constraint horizontal A329.centre A308.centre
  constraint horizontal A306.centre A332.centre
  constraint vertical A319.centre A341.centre
  constraint vertical A319.centre A335.centre
  constraint horizontal A323.centre A335.centre
  constraint horizontal A338.centre A319.centre
  constraint vertical A307.centre A318.centre
  constraint vertical A318.centre A330.centre
  constraint horizontal A325.centre A330.centre
  constraint horizontal A309.centre A318.centre
  constraint vertical A337.centre A314.centre
  constraint vertical A337.centre A322.centre
  constraint horizontal A313.centre A322.centre
  constraint horizontal A337.centre A334.centre
  constraint vertical A339.centre A336.centre
  constraint vertical A339.centre A321.centre
  constraint horizontal A321.centre A317.centre
  constraint horizontal A324.centre A339.centre
  constraint vertical A326.centre A310.centre
  constraint vertical A326.centre A311.centre
  constraint horizontal A316.centre A311.centre
  constraint horizontal A327.centre A326.centre
  constraint horizontal L38
  constraint vertical L39
  constraint horizontal L37
  constraint vertical L40
  measures "d1" diameter of A0
  measures "d2" diameter of A1
  measures "d4" diameter of A2
  measures "d5" diameter of A3
  measures "d6" diameter of A4
  measures "d7" diameter of A5
  measures "d8" distance of A0.centre A1.centre
  measures "d9" distance of A0.centre A2.centre
  measures "d10" distance of A2.centre A4.centre
  measures "d11" diameter of A6
  measures "d12" diameter of A7
  measures "d13" diameter of A9
  measures "d14" diameter of A8
  measures "d15" diameter of A11
  measures "d16" diameter of A10
  measures "d17" distance of A7.centre A6.centre
  measures "d18" distance of A9.centre A6.centre
  measures "d19" distance of A9.centre A11.centre
  measures "d20" diameter of A12
  measures "d21" diameter of A14
  measures "d22" diameter of A15
  measures "d23" diameter of A13
  measures "d24" diameter of A16
  measures "d25" diameter of A17
  measures "d26" distance of A14.centre A12.centre
  measures "d27" distance of A15.centre A12.centre
  measures "d28" distance of A15.centre A16.centre
  measures "d29" horizontal distance of A1.centre A6.centre
  measures "d30" horizontal distance of A7.centre A12.centre
  measures "d31" diameter of A18
  measures "d32" diameter of A19
  measures "d33" diameter of A23
  measures "d34" diameter of A20
  measures "d35" diameter of A30
  measures "d36" diameter of A25
  measures "d37" distance of A19.centre A18.centre
  measures "d38" distance of A23.centre A18.centre
  measures "d39" distance of A23.centre A30.centre
  measures "d40" diameter of A22
  measures "d41" diameter of A24
  measures "d42" diameter of A21
  measures "d43" diameter of A29
  measures "d44" diameter of A31
  measures "d45" diameter of A28
  measures "d46" distance of A24.centre A22.centre
  measures "d47" distance of A21.centre A22.centre
  measures "d48" distance of A21.centre A31.centre